CN06GPSholdercap (Autodesk Fusion 360 design; units mm, degrees)
Autodesk Fusion 360 part; units mm, degrees
sketch "Sketch1" plane through (0, 0, 0) normal (0, 0, 1) x (1, 0, 0)
  line L0 (18.8, 16.3) -> (-18.8, 16.3)
  line L1 (-18.8, 16.3) -> (-18.8, -16.3)
  line L2 (-18.8, -16.3) -> (18.8, -16.3)
  line L3 (18.8, -16.3) -> (18.8, 16.3)
  line L4 (18.8, 16.3) -> (-18.8, -16.3) construction
  line L5 (-18.8, 16.3) -> (18.8, -16.3) construction
  line L6 (-17, 14.5) -> (-17, -14.5)
  line L7 (-17, -14.5) -> (17, -14.5)
  line L8 (17, -14.5) -> (17, 14.5)
  line L9 (17, 14.5) -> (-17, 14.5)
  line L10 (-17, -14.5) -> (-15.8, -14.5)
  line L11 (-15.8, -14.5) -> (-15.8, -13.3)
  line L12 (-15.8, -13.3) -> (-17, -13.3)
  line L13 (-17, -13.3) -> (-17, -14.5)
  line L14 (-17, 14.5) -> (-15.8, 14.5)
  line L15 (-15.8, 14.5) -> (-15.8, 13.3)
  line L16 (-15.8, 13.3) -> (-17, 13.3)
  line L17 (-17, 13.3) -> (-17, 14.5)
  line L18 (17, -14.5) -> (13.8, -14.5)
  line L19 (13.8, -14.5) -> (13.8, -11.3)
  line L20 (13.8, -11.3) -> (17, -11.3)
  line L21 (17, -11.3) -> (17, -14.5)
  line L22 (17, 14.5) -> (13.8, 14.5)
  line L23 (13.8, 14.5) -> (13.8, 11.3)
  line L24 (13.8, 11.3) -> (17, 11.3)
  line L25 (17, 11.3) -> (17, 14.5)
  dimension "d1" = 37.6
  dimension "d2" = 32.6
  dimension "d55" = -1.8
  dimension "d73" = 1.2
  dimension "d74" = 1.2
  dimension "d75" = 1.2
  dimension "d76" = 1.2
  dimension "d77" = 3.2
  dimension "d78" = 3.2
  dimension "d79" = 3.2
  dimension "d80" = 3.2
  constraint horizontal L0
  constraint perpendicular L0 L1
  constraint parallel L0 L2
  constraint parallel L1 L3
  constraint coincident L4 origin
  constraint coincident L5 origin
  constraint horizontal L10
  constraint vertical L11
  constraint horizontal L12
  constraint vertical L13
  constraint horizontal L14
  constraint vertical L15
  constraint horizontal L16
  constraint vertical L17
  constraint horizontal L18
  constraint vertical L19
  constraint horizontal L20
  constraint vertical L21
  constraint horizontal L22
  constraint vertical L23
  constraint horizontal L24
  constraint vertical L25
  measures "d1" distance of L1.end L2.end
  measures "d2" distance of L0.end L1.end
  measures "d73" distance of L6.end L10.end
  measures "d74" distance of L6.end L12.end
  measures "d75" distance of L6.start L14.end
  measures "d76" distance of L6.start L16.end
  measures "d77" distance of L7.end L18.end
  measures "d78" distance of L7.end L20.end
  measures "d79" distance of L8.end L22.end
  measures "d80" distance of L8.end L24.end
extrude "Extrude9" add sketch "Sketch1" along normal blind 0.4 contours L0 L1 L2 L3 | L6 L9 L14 L15 L16 L17 | L6 L7 L8 L9 L11 L12 L15 L16 L19 L20 L23 L24 | L6 L7 L10 L11 L12 L13 | L8 L9 L22 L23 L24 L25 | L7 L8 L18 L19 L20 L21 picked at (4.6, -15.7) picked at (-16.2, 14.1) picked at (-5.9333, -3.7667) picked at (-16.2, -14.1) picked at (14.8667, 12.3667) picked at (14.8667, -12.3667) makes body 1
extrude "Extrude10" add sketch "Sketch1" against normal blind 5 separate body contours L0 L1 L2 L3 picked at (4.6, -15.7) makes body 2
extrude "Extrude13" add sketch "Sketch1" against normal blind 6.2 contours L7 L8 L18 L19 L20 L21 picked at (14.8667, -12.3667) bodies 1 2
extrude "Extrude14" add sketch "Sketch1" against normal blind 6.2 contours L8 L9 L22 L23 L24 L25 picked at (14.8667, 12.3667) bodies 1
extrude "Extrude15" add sketch "Sketch1" against normal blind 6.2 contours L6 L9 L14 L15 L16 L17 picked at (-16.2, 14.1) bodies 1
extrude "Extrude16" add sketch "Sketch1" against normal blind 6.2 contours L6 L7 L10 L11 L12 L13 picked at (-16.2, -14.1) bodies 1
fillet "Fillet10" radius 1 4 edges at (18.8, 16.3, -2.3) (-18.8, -16.3, -2.3) (18.8, -16.3, -2.3) (-18.8, 16.3, -2.3) on bodies 1
fillet "Fillet11" radius 0.5 4 edges at (-17, 14.5, -5.6) (-17, -14.5, -5.6) (17, -14.5, -5.6) (17, 14.5, -5.6) on bodies 1
fillet "Fillet12" radius 2 1 faces at (-5.9333, -5.4333, 0.4) on bodies 1
sketch "Sketch8" plane through (0, 0, 0) normal (1, 0, 0) x (0, 1, 0)
ref_plane "WorkPlane4" through (-18.8, 0, -3.3) normal (-1, 0, 0) x (0, -1, 0)
sketch "Sketch9" plane through (-18.8, 0, -3.3) normal (-1, 0, 0) x (0, 1, 0)
  line L0 (6.447, 1.3086) -> (6.447, -1.0914)
  line L1 (6.447, -1.0914) -> (6.1294, -1.0914)
  line L2 (6.1294, -1.0914) -> (6.1294, 1.3086)
  line L3 (6.1294, 1.3086) -> (6.447, 1.3086)
  line L4 (5.5728, 1.3086) -> (5.5728, -1.0914)
  line L5 (5.5728, -1.0914) -> (5.247, -1.0914)
  line L6 (5.247, -1.0914) -> (3.9864, 0.7929)
  line L7 (3.9864, 0.7929) -> (3.9864, -1.0914)
  line L8 (3.9864, -1.0914) -> (3.6819, -1.0914)
  line L9 (3.6819, -1.0914) -> (3.6819, 1.3086)
  line L10 (3.6819, 1.3086) -> (4.0077, 1.3086)
  line L11 (4.0077, 1.3086) -> (5.2683, -0.5774)
  line L12 (5.2683, -0.5774) -> (5.2683, 1.3086)
  line L13 (5.2683, 1.3086) -> (5.5728, 1.3086)
  line L14 (3.2661, 0.675) -> (2.9714, 0.6357)
  spline S0 degree 3 poles (2.9714, 0.6357) (2.9545, 0.7105) (2.924, 0.8444) (2.8371, 0.95) (2.7987, 0.9967) knots 0 0 0 0 0.022613 0.040507 0.040507 0.040507 0.040507
  spline S1 degree 3 poles (2.7987, 0.9967) (2.7554, 1.0289) (2.6671, 1.0945) (2.5574, 1.1029) (2.5016, 1.1072) knots 0 0 0 0 0.015864 0.032285 0.032285 0.032285 0.032285
  spline S2 degree 3 poles (2.5016, 1.1072) (2.4351, 1.1014) (2.3031, 1.0898) (2.2011, 1.0052) (2.1504, 0.9631) knots 0 0 0 0 0.01951 0.038768 0.038768 0.038768 0.038768
  spline S3 degree 3 poles (2.1504, 0.9631) (2.1087, 0.9118) (2.024, 0.8078) (2.0128, 0.674) (2.0072, 0.6063) knots 0 0 0 0 0.019377 0.039265 0.039265 0.039265 0.039265
  spline S4 degree 3 poles (2.0072, 0.6063) (2.0122, 0.5421) (2.0219, 0.4167) (2.1011, 0.3191) (2.1398, 0.2715) knots 0 0 0 0 0.018814 0.036778 0.036778 0.036778 0.036778
  spline S5 degree 3 poles (2.1398, 0.2715) (2.1878, 0.233) (2.2864, 0.1542) (2.4124, 0.1446) (2.477, 0.1397) knots 0 0 0 0 0.018015 0.036967 0.036967 0.036967 0.036967
  spline S6 degree 3 poles (2.477, 0.1397) (2.5084, 0.1415) (2.5787, 0.1457) (2.6471, 0.1629) (2.6849, 0.1724) knots 0 0 0 0 0.009408 0.021088 0.021088 0.021088 0.021088
  line L15 (2.6849, 0.1724) -> (2.6522, -0.0862)
  spline S7 degree 3 poles (2.6522, -0.0862) (2.6433, -0.0853) (2.6276, -0.0836) (2.6117, -0.0832) (2.6047, -0.083) knots 0 0 0 0 0.002672 0.004761 0.004761 0.004761 0.004761
  spline S8 degree 3 poles (2.6047, -0.083) (2.5439, -0.0869) (2.4236, -0.0945) (2.318, -0.1525) (2.2658, -0.1812) knots 0 0 0 0 0.018053 0.03567 0.03567 0.03567 0.03567
  spline S9 degree 3 poles (2.2658, -0.1812) (2.2219, -0.2196) (2.1306, -0.2995) (2.1205, -0.421) (2.1152, -0.4841) knots 0 0 0 0 0.016835 0.035033 0.035033 0.035033 0.035033
  spline S10 degree 3 poles (2.1152, -0.4841) (2.1195, -0.5355) (2.1279, -0.6366) (2.1929, -0.7143) (2.2249, -0.7525) knots 0 0 0 0 0.015067 0.029644 0.029644 0.029644 0.029644
  spline S11 degree 3 poles (2.2249, -0.7525) (2.2651, -0.7836) (2.3484, -0.8479) (2.4537, -0.8552) (2.5081, -0.859) knots 0 0 0 0 0.014885 0.030865 0.030865 0.030865 0.030865
  spline S12 degree 3 poles (2.5081, -0.859) (2.5626, -0.8549) (2.6688, -0.847) (2.7534, -0.7824) (2.7946, -0.7509) knots 0 0 0 0 0.015987 0.031215 0.031215 0.031215 0.031215
  spline S13 degree 3 poles (2.7946, -0.7509) (2.8298, -0.7077) (2.9069, -0.6128) (2.9296, -0.4923) (2.942, -0.4268) knots 0 0 0 0 0.016463 0.036106 0.036106 0.036106 0.036106
  line L16 (2.942, -0.4268) -> (3.2367, -0.4791)
  spline S14 degree 3 poles (3.2367, -0.4791) (3.2146, -0.5709) (3.1726, -0.7457) (3.0496, -0.8763) (2.9911, -0.9384) knots 0 0 0 0 0.027742 0.052885 0.052885 0.052885 0.052885
  spline S15 degree 3 poles (2.9911, -0.9384) (2.9218, -0.9859) (2.7784, -1.0842) (2.6046, -1.0954) (2.5147, -1.1012) knots 0 0 0 0 0.024717 0.051185 0.051185 0.051185 0.051185
  spline S16 degree 3 poles (2.5147, -1.1012) (2.4509, -1.0979) (2.3252, -1.0914) (2.2098, -1.0415) (2.1529, -1.0169) knots 0 0 0 0 0.018985 0.037416 0.037416 0.037416 0.037416
  spline S17 degree 3 poles (2.1529, -1.0169) (2.1014, -0.9869) (2.0007, -0.9281) (1.933, -0.8332) (1.9, -0.7869) knots 0 0 0 0 0.017669 0.034536 0.034536 0.034536 0.034536
  spline S18 degree 3 poles (1.9, -0.7869) (1.8744, -0.7379) (1.8238, -0.6408) (1.8162, -0.5316) (1.8124, -0.4775) knots 0 0 0 0 0.016394 0.032465 0.032465 0.032465 0.032465
  spline S19 degree 3 poles (1.8124, -0.4775) (1.8158, -0.4269) (1.8226, -0.3263) (1.8715, -0.2381) (1.8959, -0.1943) knots 0 0 0 0 0.015003 0.029853 0.029853 0.029853 0.029853
  spline S20 degree 3 poles (1.8959, -0.1943) (1.9281, -0.1534) (1.9957, -0.0679) (2.0925, -0.0176) (2.1431, 0.0087) knots 0 0 0 0 0.015445 0.032313 0.032313 0.032313 0.032313
  spline S21 degree 3 poles (2.1431, 0.0087) (2.0768, 0.0286) (1.9482, 0.0672) (1.8567, 0.1651) (1.8124, 0.2125) knots 0 0 0 0 0.020361 0.03947 0.03947 0.03947 0.03947
  spline S22 degree 3 poles (1.8124, 0.2125) (1.778, 0.269) (1.7058, 0.3878) (1.6984, 0.5268) (1.6945, 0.5997) knots 0 0 0 0 0.01953 0.041036 0.041036 0.041036 0.041036
  spline S23 degree 3 poles (1.6945, 0.5997) (1.7041, 0.7006) (1.7234, 0.9027) (1.8568, 1.0559) (1.9237, 1.1326) knots 0 0 0 0 0.029598 0.059322 0.059322 0.059322 0.059322
  spline S24 degree 3 poles (1.9237, 1.1326) (2.0067, 1.1963) (2.1775, 1.3275) (2.3926, 1.3431) (2.5032, 1.3511) knots 0 0 0 0 0.030692 0.06316 0.06316 0.06316 0.06316
  spline S25 degree 3 poles (2.5032, 1.3511) (2.6029, 1.3444) (2.7959, 1.3312) (2.9523, 1.2178) (3.0279, 1.1629) knots 0 0 0 0 0.029296 0.056758 0.056758 0.056758 0.056758
  spline S26 degree 3 poles (3.0279, 1.1629) (3.0901, 1.0946) (3.2169, 0.9553) (3.2495, 0.7696) (3.2661, 0.675) knots 0 0 0 0 0.027123 0.055296 0.055296 0.055296 0.055296
  line L17 (1.5472, 1.3086) -> (0.6255, -1.0914)
  line L18 (0.6255, -1.0914) -> (0.2833, -1.0914)
  line L19 (0.2833, -1.0914) -> (-0.699, 1.3086)
  line L20 (-0.699, 1.3086) -> (-0.3372, 1.3086)
  line L21 (-0.3372, 1.3086) -> (-0.0572, 0.5817)
  line L22 (-0.0572, 0.5817) -> (0.9463, 0.5817)
  line L23 (0.9463, 0.5817) -> (1.2099, 1.3086)
  line L24 (1.2099, 1.3086) -> (1.5472, 1.3086)
  line L25 (0.8547, 0.323) -> (0.041, 0.323)
  line L26 (0.041, 0.323) -> (0.2915, -0.3416)
  spline S27 degree 3 poles (0.2915, -0.3416) (0.3258, -0.4332) (0.3874, -0.5975) (0.4389, -0.7651) (0.4618, -0.8393) knots 0 0 0 0 0.029337 0.05261 0.05261 0.05261 0.05261
  spline S28 degree 3 poles (0.4618, -0.8393) (0.4787, -0.7622) (0.5129, -0.6069) (0.5649, -0.4566) (0.5911, -0.3809) knots 0 0 0 0 0.023656 0.047665 0.047665 0.047665 0.047665
  line L27 (0.5911, -0.3809) -> (0.8547, 0.323)
  spline S29 degree 3 poles (-2.7715, 1.0515) (-2.8411, 1.0978) (-2.9705, 1.184) (-3.1132, 1.2457) (-3.1792, 1.2742) knots 0 0 0 0 0.024998 0.046531 0.046531 0.046531 0.046531
  line L28 (-3.1792, 1.2742) -> (-3.0859, 1.4952)
  spline S30 degree 3 poles (-3.0859, 1.4952) (-2.998, 1.4582) (-2.8142, 1.3809) (-2.6539, 1.2624) (-2.5702, 1.2005) knots 0 0 0 0 0.028491 0.059583 0.059583 0.059583 0.059583
  spline S31 degree 3 poles (-2.5702, 1.2005) (-2.4782, 1.244) (-2.2915, 1.3321) (-2.0853, 1.3437) (-1.9808, 1.3495) knots 0 0 0 0 0.030218 0.061301 0.061301 0.061301 0.061301
  spline S32 degree 3 poles (-1.9808, 1.3495) (-1.8754, 1.3433) (-1.6676, 1.3312) (-1.4815, 1.2382) (-1.3898, 1.1923) knots 0 0 0 0 0.031312 0.061724 0.061724 0.061724 0.061724
  spline S33 degree 3 poles (-1.3898, 1.1923) (-1.3063, 1.1342) (-1.1377, 1.0169) (-1.0338, 0.8397) (-0.9814, 0.7503) knots 0 0 0 0 0.030141 0.060826 0.060826 0.060826 0.060826
  spline S34 degree 3 poles (-0.9814, 0.7503) (-0.9396, 0.6507) (-0.8535, 0.4455) (-0.8433, 0.2231) (-0.8381, 0.1086) knots 0 0 0 0 0.032136 0.066212 0.066212 0.066212 0.066212
  spline S35 degree 3 poles (-0.8381, 0.1086) (-0.8435, -0.006) (-0.8541, -0.23) (-0.9402, -0.437) (-0.9822, -0.5381) knots 0 0 0 0 0.03412 0.0667 0.0667 0.0667 0.0667
  spline S36 degree 3 poles (-0.9822, -0.5381) (-1.0346, -0.629) (-1.1377, -0.808) (-1.3083, -0.9244) (-1.3923, -0.9817) knots 0 0 0 0 0.031036 0.061113 0.061113 0.061113 0.061113
  spline S37 degree 3 poles (-1.3923, -0.9817) (-1.4846, -1.0261) (-1.6726, -1.1166) (-1.8812, -1.1281) (-1.9874, -1.134) knots 0 0 0 0 0.030404 0.061965 0.061965 0.061965 0.061965
  spline S38 degree 3 poles (-1.9874, -1.134) (-2.0946, -1.1279) (-2.3051, -1.1159) (-2.4939, -1.0221) (-2.5865, -0.976) knots 0 0 0 0 0.031842 0.062543 0.062543 0.062543 0.062543
  spline S39 degree 3 poles (-2.5865, -0.976) (-2.6703, -0.9178) (-2.8388, -0.8008) (-2.9417, -0.6233) (-2.9934, -0.534) knots 0 0 0 0 0.030198 0.060735 0.060735 0.060735 0.060735
  spline S40 degree 3 poles (-2.9934, -0.534) (-3.0342, -0.4345) (-3.1184, -0.2292) (-3.1283, -0.0074) (-3.1333, 0.1069) knots 0 0 0 0 0.031996 0.066044 0.066044 0.066044 0.066044
  spline S41 degree 3 poles (-3.1333, 0.1069) (-3.1302, 0.2015) (-3.1242, 0.3833) (-3.0695, 0.5566) (-3.0433, 0.6398) knots 0 0 0 0 0.028228 0.054269 0.054269 0.054269 0.054269
  spline S42 degree 3 poles (-3.0433, 0.6398) (-3.0095, 0.7161) (-2.9419, 0.8685) (-2.8283, 0.9906) (-2.7715, 1.0515) knots 0 0 0 0 0.024839 0.049641 0.049641 0.049641 0.049641
  spline S43 degree 3 poles (-2.0725, 0.6455) (-2.1584, 0.6729) (-2.3221, 0.725) (-2.4603, 0.8266) (-2.526, 0.8747) knots 0 0 0 0 0.026855 0.051113 0.051113 0.051113 0.051113
  spline S44 degree 3 poles (-2.526, 0.8747) (-2.6075, 0.7726) (-2.7856, 0.5494) (-2.7988, 0.2626) (-2.8059, 0.1069) knots 0 0 0 0 0.038243 0.083602 0.083602 0.083602 0.083602
  spline S45 degree 3 poles (-2.8059, 0.1069) (-2.8027, 0.0149) (-2.7966, -0.1602) (-2.7357, -0.3243) (-2.7069, -0.4022) knots 0 0 0 0 0.027411 0.052167 0.052167 0.052167 0.052167
  spline S46 degree 3 poles (-2.7069, -0.4022) (-2.6705, -0.4704) (-2.599, -0.6047) (-2.4771, -0.6955) (-2.4171, -0.7403) knots 0 0 0 0 0.022863 0.045019 0.045019 0.045019 0.045019
  spline S47 degree 3 poles (-2.4171, -0.7403) (-2.3511, -0.7754) (-2.2171, -0.8465) (-2.0657, -0.8559) (-1.989, -0.8606) knots 0 0 0 0 0.02216 0.044931 0.044931 0.044931 0.044931
  spline S48 degree 3 poles (-1.989, -0.8606) (-1.8762, -0.8511) (-1.6539, -0.8323) (-1.4836, -0.6884) (-1.3996, -0.6175) knots 0 0 0 0 0.03306 0.065177 0.065177 0.065177 0.065177
  spline S49 degree 3 poles (-1.3996, -0.6175) (-1.3315, -0.5198) (-1.1804, -0.3029) (-1.1708, -0.0373) (-1.1655, 0.1086) knots 0 0 0 0 0.035026 0.077727 0.077727 0.077727 0.077727
  spline S50 degree 3 poles (-1.1655, 0.1086) (-1.1713, 0.2511) (-1.182, 0.5133) (-1.3297, 0.7289) (-1.3972, 0.8273) knots 0 0 0 0 0.041781 0.076875 0.076875 0.076875 0.076875
  spline S51 degree 3 poles (-1.3972, 0.8273) (-1.4806, 0.9003) (-1.6502, 1.0487) (-1.8749, 1.068) (-1.989, 1.0777) knots 0 0 0 0 0.032384 0.06578 0.06578 0.06578 0.06578
  spline S52 degree 3 poles (-1.989, 1.0777) (-2.0447, 1.0752) (-2.1549, 1.0701) (-2.2586, 1.0325) (-2.3099, 1.0139) knots 0 0 0 0 0.016612 0.032885 0.032885 0.032885 0.032885
  spline S53 degree 3 poles (-2.3099, 1.0139) (-2.2598, 0.9841) (-2.1608, 0.9251) (-2.0502, 0.8925) (-1.9955, 0.8764) knots 0 0 0 0 0.017397 0.03443 0.03443 0.03443 0.03443
  line L29 (-1.9955, 0.8764) -> (-2.0725, 0.6455)
  line L30 (-3.5475, 1.3086) -> (-3.5475, -1.0914)
  line L31 (-3.5475, -1.0914) -> (-3.8651, -1.0914)
  line L32 (-3.8651, -1.0914) -> (-3.8651, 0.0988)
  line L33 (-3.8651, 0.0988) -> (-5.0569, -1.0914)
  line L34 (-5.0569, -1.0914) -> (-5.4875, -1.0914)
  line L35 (-5.4875, -1.0914) -> (-4.4807, -0.119)
  line L36 (-4.4807, -0.119) -> (-5.5317, 1.3086)
  line L37 (-5.5317, 1.3086) -> (-5.1126, 1.3086)
  line L38 (-5.1126, 1.3086) -> (-4.258, 0.0938)
  line L39 (-4.258, 0.0938) -> (-3.8651, 0.4769)
  line L40 (-3.8651, 0.4769) -> (-3.8651, 1.3086)
  line L41 (-3.8651, 1.3086) -> (-3.5475, 1.3086)
extrude "Extrude17" cut sketch "Sketch9" against normal blind 0.4 contours L0 L1 L2 L3 | L4 L5 L6 L7 L8 L9 L10 L11 L12 L13 | L14 S0 S1 S2 S3 S4 S5 S6 L15 S8 S9 S10 S11 S12 S13 L16 S14 S15 S16 S17 S18 S19 S20 S21 S22 S23 S24 S25 S26 | L17 L18 L19 L20 L21 L22 L23 L24 | S29 L28 S30 S31 S32 S33 S34 S35 S36 S37 S38 S39 S40 S41 S42 | L30 L31 L32 L33 L34 L35 L36 L37 L38 L39 L40 L41 picked at (6.2353, 0.5086) picked at (3.7834, 0.3367) picked at (2.2825, 0.0133) picked at (-0.1249, 0.1801) picked at (-0.9587, -0.0408) picked at (-5.0417, 0.8327) bodies 1
